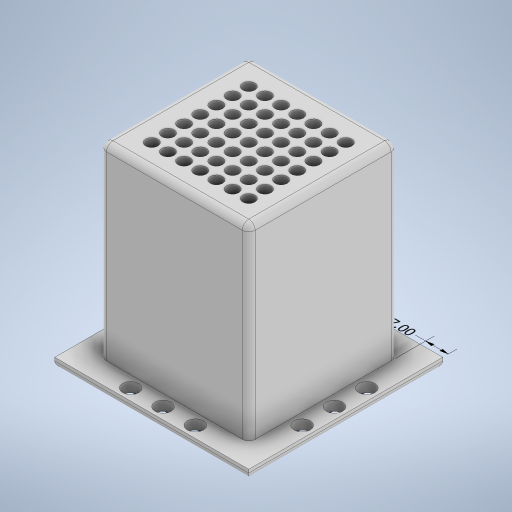
# Autodesk Inventor part: cache-suspensions
Saved by Autodesk Inventor 2023 (Build 270158000, 158)
## iProperties
Created: 2023-02-20
Part Number: cache-suspensions
Material: Générique
Document SubType Name: Modeling
Designer: pined
Density: 1 g/cm^3
Appearance: Par défaut
Author: pined
Autodesk Inventor part; units mm, degrees
ref_plane "YZ Plane" through (0, 0, 0) normal (1, 0, 0) x (0, 1, 0)
ref_plane "XZ Plane" through (0, 0, 0) normal (0, 1, 0) x (-1, 0, 0)
ref_plane "XY Plane" through (0, 0, 0) normal (0, 0, 1) x (1, 0, 0)
sketch "Esquisse1" plane through (0, 0, 0) normal (0, 1, 0) x (-1, 0, 0)
  line L0 (18.004, 21.8884) -> (-22.996, 21.8884)
  line L1 (-22.996, 21.8884) -> (-22.996, -19.1116)
  line L2 (-22.996, -19.1116) -> (18.004, -19.1116)
  line L3 (18.004, -19.1116) -> (18.004, 21.8884)
  line L4 (19.004, 22.8884) -> (-23.996, 22.8884)
  line L5 (-23.996, 22.8884) -> (-23.996, -20.1116)
  line L6 (-23.996, -20.1116) -> (19.004, -20.1116)
  line L7 (19.004, -20.1116) -> (19.004, 22.8884)
  point P0 (0, 0)
  dimension "d0" = 41
  dimension "d1" = 41
  dimension "d2" = 43
  dimension "d3" = 43
  dimension "d4" = 1
  dimension "d5" = 1
  constraints: 16 end point, 4 parallel, 2 horizontal, 2 perpendicular
  measures "d0" distance of L2.end L0.start
  measures "d1" distance of L0.start L0.end
  measures "d2" distance of L6.end L4.start
  measures "d3" distance of L5.end L6.end
  measures "d4" distance between parallel lines of L3 L7
  measures "d5" distance between parallel lines of L2 L6
extrude "Extrusion1" add sketch "Esquisse1" along normal blind 3
sketch "Esquisse2" plane through (0, 3, 0) normal (0, 1, 0) x (1, 0, 0)
  line L0 (-27.504, -31.3884) -> (32.496, -31.3884)
  line L1 (32.496, -31.3884) -> (32.496, 28.6116)
  line L2 (32.496, 28.6116) -> (-27.504, 28.6116)
  line L3 (-27.504, 28.6116) -> (-27.504, -31.3884)
  line L4 (-19.004, -22.8884) -> (23.996, -22.8884) projected
  line L5 (-19.004, 20.1116) -> (-19.004, -22.8884) projected
  line L6 (22.996, 19.1116) -> (22.996, -21.8884) projected
  line L7 (-18.004, -21.8884) -> (22.996, -21.8884)
  line L8 (22.996, -21.8884) -> (22.996, 19.1116)
  line L9 (22.996, 19.1116) -> (-18.004, 19.1116)
  line L10 (-18.004, 19.1116) -> (-18.004, -21.8884)
  point P0 (0, 0)
  point P1 (22.996, -21.8884)
  dimension "d8" = 60
  dimension "d9" = 60
  dimension "d10" = 8.5
  dimension "d11" = 8.5
  constraints: 16 end point, 4 parallel, 2 horizontal, 2 perpendicular
  measures "d8" distance of L0.start L0.end
  measures "d9" distance of L2.end L0.start
  measures "d10" distance between parallel lines of L0 L4
  measures "d11" distance between parallel lines of L5 L3
extrude "Extrusion2" add sketch "Esquisse2" along normal blind 3
sketch "Esquisse3" plane through (0, 6, 0) normal (0, 1, 0) x (1, 0, 0)
  line L0 (-20.504, -24.3884) -> (25.496, -24.3884)
  line L1 (25.496, -24.3884) -> (25.496, 21.6116)
  line L2 (25.496, 21.6116) -> (-20.504, 21.6116)
  line L3 (-20.504, 21.6116) -> (-20.504, -24.3884)
  line L4 (22.996, -21.8884) -> (-18.004, -21.8884) projected
  line L5 (-18.004, -21.8884) -> (-18.004, 19.1116) projected
  line L6 (-18.004, -21.8884) -> (22.996, -21.8884)
  line L7 (22.996, -21.8884) -> (22.996, 19.1116)
  line L8 (22.996, 19.1116) -> (-18.004, 19.1116)
  line L9 (-18.004, 19.1116) -> (-18.004, -21.8884)
  point P0 (0, 0)
  dimension "d14" = 46
  dimension "d15" = 46
  dimension "d16" = 2.5
  dimension "d17" = 2.5
  constraints: 16 end point, 4 parallel, 2 horizontal, 2 perpendicular
  measures "d14" distance of L2.end L0.start
  measures "d15" distance of L0.start L0.end
  measures "d16" distance between parallel lines of L4 L0
  measures "d17" distance between parallel lines of L5 L3
extrude "Extrusion3" add sketch "Esquisse3" along normal blind 55
sketch "Esquisse4" plane through (0, 61, 0) normal (0, 1, 0) x (1, 0, 0)
  line L0 (25.496, -24.3884) -> (25.496, 21.6116) projected
  line L1 (-20.504, 21.6116) -> (25.496, 21.6116)
  line L2 (25.496, 21.6116) -> (25.496, -24.3884)
  line L3 (25.496, -24.3884) -> (-20.504, -24.3884)
  line L4 (-20.504, -24.3884) -> (-20.504, 21.6116)
  point P0 (0, 0)
  constraints: 8 end point, 2 parallel, 1 horizontal, 1 perpendicular
extrude "Extrusion4" add sketch "Esquisse4" along normal blind 3
sketch "Esquisse5" plane through (0, 6, 0) normal (0, 1, 0) x (1, 0, 0)
  circle A0 centre (28.996, -1.3884) radius 2.5
  line L0 (32.496, -31.3884) -> (32.496, 28.6116) projected
  circle A1 centre (28.996, 8.6116) radius 2.5
  circle A2 centre (28.996, -11.3884) radius 2.5
  line L1 (32.496, 28.6116) -> (-27.504, 28.6116) projected
  line L2 (2.496, 28.6116) -> (2.496, -31.3884)
  line L3 (-27.504, -31.3884) -> (32.496, -31.3884) projected
  line L4 (32.496, -1.3884) -> (-27.504, -1.3884)
  line L5 (-27.504, 28.6116) -> (-27.504, -31.3884) projected
  circle A3 centre (-24.004, -1.3884) radius 2.5
  circle A4 centre (-24.004, 8.6116) radius 2.5
  circle A5 centre (-24.004, -11.3884) radius 2.5
  circle A6 centre (2.496, -27.8884) radius 2.5
  circle A7 centre (12.496, -27.8884) radius 2.5
  circle A8 centre (-7.504, -27.8884) radius 2.5
  circle A9 centre (2.496, 25.1116) radius 2.5
  circle A10 centre (12.496, 25.1116) radius 2.5
  circle A11 centre (-7.504, 25.1116) radius 2.5
  point P0 (0, 0)
  dimension "d32" = 10
  dimension "d25" = 5
  dimension "d26" = 3.5
  dimension "d29" = 10
  dimension "d36" = 10
  dimension "d41" = 0
  dimension "d42" = 5
  dimension "d43" = 3.5
  dimension "d46" = 10
  dimension "d53" = 10
  constraints: 12 centre point, 6 symmetric about line, 4 end point, 4 midpoint, 2 horizontal, 2 vertical, 1 point on line, 14 other
  measures "d25" diameter of A0
  measures "d26" distance from line of A0.centre L0
  measures "d29" distance of A0.centre A1.centre
  measures "d36" distance of A0.centre A2.centre
  measures "d41" distance from line of L4 A0.centre
  measures "d42" diameter of A6
  measures "d43" distance from line of L3 A6.centre
  measures "d46" distance of A6.centre A7.centre
  measures "d53" distance of A6.centre A8.centre
extrude "Extrusion5" cut sketch "Esquisse5" against normal through all contours L4 A0 | A0 L4 | A9 L2 | L2 A9 | A6 L2 | L2 A6 | A3 L4 | L4 A3 | A1 | A2 | A4 | A5 | A7 | A8 | A10 | A11
fillet "Congé1" radius 2 20 edges at (25.496, 35, -21.6116) (25.496, 35, 24.3884) (25.496, 64, 1.3884) (-20.504, 35, 24.3884) (2.496, 64, 24.3884) (-20.504, 64, 1.3884) (2.496, 64, -21.6116) (-20.504, 35, -21.6116) (-27.504, 3, 1.3884) (2.496, 3, -28.6116) (32.496, 3, 1.3884) (2.496, 3, 31.3884) (-18.004, 61, 1.3884) (2.496, 61, -19.1116) (22.996, 61, 1.3884) (2.496, 61, 21.8884) (-18.004, 30.5, 21.8884) (22.996, 30.5, 21.8884) (22.996, 30.5, -19.1116) (-18.004, 30.5, -19.1116)
sketch "Esquisse6" plane through (0, 61, 0) normal (0, -1, 0) x (1, 0, 0)
  circle A0 centre (17.996, 16.8884) radius 1.9
  line L0 (-16.004, 19.8884) -> (20.996, 19.8884) projected
  line L1 (20.996, 19.8884) -> (20.996, -17.1116) projected
  point P0 (0, 0)
  dimension "d61" = 3.8
  dimension "d62" = 3
  dimension "d63" = 3
  constraints: 1 centre point
  measures "d61" diameter of A0
  measures "d62" distance from line of L0 A0.centre
  measures "d63" distance from line of A0.centre L1
extrude "Extrusion6" cut sketch "Esquisse6" against normal through all
pattern_linear "Réseau rectangulaire1" count 7 spacing 5 along (0, 0, -1) count 7 spacing 5 along (-1, 0, 0) of "Extrusion6"
sketch "Esquisse7" plane through (0, 0, 0) normal (0, -1, 0) x (1, 0, 0)
  line L0 (-18.504, -19.6116) -> (-20.504, -19.6116) projected
  line L1 (23.496, 22.3884) -> (-18.504, 22.3884) projected
  line L2 (-18.504, -19.6116) -> (23.496, -19.6116)
  line L3 (23.496, -19.6116) -> (23.496, 22.3884)
  line L4 (23.496, 22.3884) -> (-18.504, 22.3884)
  line L5 (-18.504, 22.3884) -> (-18.504, -19.6116)
  line L6 (23.996, 22.8884) -> (23.996, -20.1116) projected
  point P0 (0, 0)
  point P1 (-18.504, 22.3884)
  dimension "d72" = 0.5
  constraints: 8 end point, 2 parallel, 1 horizontal, 1 perpendicular, 1 point on line
  measures "d72" distance between parallel lines of L6 L3
extrude "Extrusion7" cut sketch "Esquisse7" against normal up to surface (61 mm away)
